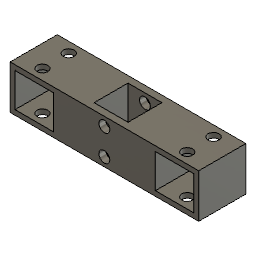
JointBar (Autodesk Fusion 360 design; units mm, degrees)
Autodesk Fusion 360 part; units mm, degrees
note: some values were not read from the file. Set by a fixed rule: which sketch regions a step uses.
sketch "Sketch3" plane through (0, 0, 18) normal (0, 0, 1) x (1, 0, 0)
  line L0 (-33.9, 6.35) -> (-19.5, 6.35) construction
  line L1 (-19.5, 6.35) -> (-19.5, -6.35) construction
  line L2 (-19.5, -6.35) -> (-33.9, -6.35) construction
  line L3 (-33.9, -6.35) -> (-33.9, 6.35) construction
  line L4 (19.5, 6.35) -> (33.9, 6.35) construction
  line L5 (33.9, 6.35) -> (33.9, -6.35) construction
  line L6 (33.9, -6.35) -> (19.5, -6.35) construction
  line L7 (19.5, -6.35) -> (19.5, 6.35) construction
  line L8 (-35.9, 8.35) -> (35.9, 8.35)
  line L9 (35.9, 8.35) -> (35.9, -8.35)
  line L10 (35.9, -8.35) -> (-35.9, -8.35)
  line L11 (-35.9, -8.35) -> (-35.9, 8.35)
  line L12 (-35.9, 8.35) -> (35.9, -8.35) construction
  line L13 (34, 6.45) -> (34, -6.45)
  line L14 (34, -6.45) -> (19.4, -6.45)
  line L15 (19.4, -6.45) -> (19.4, 6.45)
  line L16 (19.4, 6.45) -> (34, 6.45)
  line L17 (-19.4, -6.45) -> (-34, -6.45)
  line L18 (-34, -6.45) -> (-34, 6.45)
  line L19 (-34, 6.45) -> (-19.4, 6.45)
  line L20 (-19.4, 6.45) -> (-19.4, -6.45)
  dimension "d5" = 14.4
  dimension "d6" = 12.7
  dimension "d7" = 14.4
  dimension "d8" = 12.7
  dimension "d9" = 39
  dimension "d12" = 2
  dimension "d13" = 2
  dimension "d15" = 2
  dimension "d16" = 2
  constraint horizontal L0
  constraint vertical L1
  constraint horizontal L2
  constraint vertical L3
  constraint horizontal L4
  constraint vertical L5
  constraint horizontal L6
  constraint vertical L7
  constraint collinear L2 L6
  constraint vertical L11
  constraint horizontal L8
  constraint horizontal L10
  constraint vertical L9
  constraint midpoint L12 origin
  measures "d5" distance of L0.start L0.end
  measures "d6" distance of L0.start L2.end
  measures "d7" distance of L4.start L4.end
  measures "d8" distance of L4.end L5.end
  measures "d9" distance of L1 L7
  measures "d12" distance of L3 L11
  measures "d13" distance of L0 L8
  measures "d15" distance of L5 L9
  measures "d16" distance of L6 L10
extrude "Extrude3" add sketch "Sketch3" along normal blind 18
sketch "Sketch4" plane through (0, 8.35, 0) normal (0, 1, 0) x (-1, 0, 0)
  line L0 (-35.9, 18) -> (35.9, 18)
  line L1 (35.9, 18) -> (35.9, 36)
  line L2 (35.9, 36) -> (-35.9, 36)
  line L3 (-35.9, 36) -> (-35.9, 18)
  circle A0 centre (27.55, 22) radius 2.075
  circle A1 centre (27.55, 32) radius 2.075
  line L4 (35.9, 27) -> (-35.9, 27) construction
  line L5 (34, 18) -> (34, 36)
  line L6 (34, 36) -> (34, 18)
  line L7 (19.4, 18) -> (19.4, 36)
  line L8 (19.4, 36) -> (19.4, 18)
  line L9 (34, 18) -> (19.4, 18) construction
  line L10 (34, 36) -> (19.4, 36) construction
  line L11 (27.55, 18) -> (27.55, 36)
  line L12 (0, 18) -> (0, 36) construction
  circle A2 centre (-27.55, 22) radius 2.075
  circle A3 centre (-27.55, 32) radius 2.075
  line L13 (26.7, 18) -> (26.7, 36) construction
  point P0 (27.55, 18)
  point P1 (27.55, 36)
  dimension "d19" = 4.15
  dimension "d22" = 10
  dimension "d23" = 5
  dimension "d48" = 6.45
  constraint equal A0 A1
  constraint midpoint L1 L4.start
  constraint midpoint L3 L4.end
  constraint coincident L5.start L6.end
  constraint coincident L7.start L8.end
  constraint coincident L5.end L6.start
  constraint coincident L7.end L8.start
  constraint coincident P0 L11.start
  constraint coincident P1 L11.end
  constraint coincident A0.centre L11
  constraint coincident A1.centre L11
  constraint midpoint L0 L12.start
  constraint midpoint L2 L12.end
  constraint symmetric A0 L12 A2
  constraint symmetric A1 L12 A3
  constraint midpoint L9 L13.start
  constraint midpoint L10 L13.end
  constraint coincident L9 P0
  constraint coincident L10 P1
  constraint vertical L11
  measures "d19" diameter of A0
  measures "d22" distance of A0.centre A1.centre
  measures "d23" distance of A0.centre L4
  measures "d48" distance of L5 L11
extrude "Extrude4" cut sketch "Sketch4" against normal blind 16.7 contours A0 L11 | A0 L11 | A1 L11 | A1 L11 | A2 | A3
sketch "Sketch5" plane through (0, 8.35, 0) normal (0, 1, 0) x (-1, 0, 0)
  circle A0 centre (27.55, 32) radius 2.075
  circle A1 centre (27.55, 22) radius 2.075
  line L0 (-35.9, 18) -> (35.9, 18)
  line L1 (35.9, 18) -> (35.9, 36)
  line L2 (35.9, 36) -> (-35.9, 36)
  line L3 (-35.9, 36) -> (-35.9, 18)
  line L4 (35.9, 27) -> (-35.9, 27) construction
  line L5 (0, 18) -> (0, 36) construction
  line L6 (-6.35, 20.65) -> (6.35, 20.65) construction
  line L7 (6.35, 20.65) -> (6.35, 33.35) construction
  line L8 (6.35, 33.35) -> (-6.35, 33.35) construction
  line L9 (-6.35, 33.35) -> (-6.35, 20.65) construction
  line L10 (-6.35, 20.65) -> (6.35, 33.35) construction
  line L11 (6.35, 20.65) -> (-6.35, 33.35) construction
  circle A2 centre (-27.55, 22) radius 2.075
  circle A3 centre (-27.55, 32) radius 2.075
  line L12 (-6.45, 33.45) -> (-6.45, 20.55)
  line L13 (-6.45, 20.55) -> (6.45, 20.55)
  line L14 (6.45, 20.55) -> (6.45, 33.45)
  line L15 (6.45, 33.45) -> (-6.45, 33.45)
  point P0 (0, 27)
  dimension "d27" = 12.7
  dimension "d28" = 12.7
  dimension "d40" = 0.1
  constraint midpoint L1 L4.start
  constraint midpoint L3 L4.end
  constraint midpoint L0 L5.start
  constraint midpoint L2 L5.end
  constraint horizontal L6
  constraint perpendicular L6 L7
  constraint parallel L6 L8
  constraint parallel L7 L9
  constraint coincident L10 P0
  constraint coincident L11 P0
  constraint midpoint L4 P0
  measures "d27" distance of L7.end L8.end
  measures "d28" distance of L6.end L7.end
extrude "Extrude5" cut sketch "Sketch5" against normal blind 16.7 contours L12 L13 L14 L15
sketch "Sketch6" plane through (0, 0, 36) normal (0, 0, 1) x (1, 0, 0)
  line L0 (-35.9, -8.35) -> (35.9, -8.35)
  line L1 (35.9, -8.35) -> (35.9, 8.35)
  line L2 (35.9, 8.35) -> (-35.9, 8.35)
  line L3 (-35.9, 8.35) -> (-35.9, -8.35)
  line L4 (6.45, 0) -> (-6.45, 0) construction
  circle A0 centre (0, 5) radius 2.075
  circle A1 centre (0, -5) radius 2.075
  line L5 (-34, 6.45) -> (-19.4, 6.45)
  line L6 (-19.4, 6.45) -> (-19.4, -6.45)
  line L7 (-19.4, -6.45) -> (-34, -6.45)
  line L8 (-34, -6.45) -> (-34, 6.45)
  line L9 (19.4, -6.45) -> (19.4, 6.45)
  line L10 (19.4, 6.45) -> (34, 6.45)
  line L11 (34, 6.45) -> (34, -6.45)
  line L12 (34, -6.45) -> (19.4, -6.45)
  line L13 (-6.45, 8.35) -> (6.45, 8.35)
  line L14 (6.45, 8.35) -> (6.45, -8.35)
  line L15 (6.45, -8.35) -> (-6.45, -8.35)
  line L16 (-6.45, -8.35) -> (-6.45, 8.35)
  line L17 (0, 8.35) -> (0, -8.35) construction
  dimension "d31" = 4.15
  dimension "d32" = 10
  dimension "d33" = 5
  constraint midpoint L4.start L14
  constraint midpoint L4.end L16
  constraint equal A0 A1
  constraint midpoint L13 L17.start
  constraint midpoint L15 L17.end
  constraint coincident A0.centre L17
  constraint coincident A1.centre L17
  measures "d31" diameter of A0
  measures "d32" vertical distance of A0.centre A1.centre
  measures "d33" distance of L4 A0.centre
extrude "Extrude6" cut sketch "Sketch6" against normal blind 18 contours A0 | A1
equation "d5 = 12.7 mm + addl_wire_space"
equation "d7 = 12.7 mm + addl_wire_space"
equation "d19 = 4 mm + tolerance_hole"
equation "d31 = 4 mm + tolerance_hole"
equation "tolerance_bar = 0.1 mm"
equation "tolerance_hole = 0.15 mm"
equation "d38 = -tolerance_bar"
equation "d39 = -tolerance_bar"
equation "d40 = tolerance_bar"
equation "addl_wire_space = 0.9 mm + 0.8 mm"
equation "d48 = 12.7 mm / 2 + tolerance_bar"
